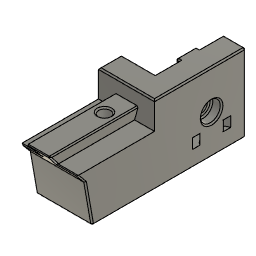
Support_arm_mount_Endcap_f360_v1 (Autodesk Fusion 360 design; units mm, degrees)
Autodesk Fusion 360 part; units mm, degrees
note: some values were not read from the file. Set by a fixed rule: which sketch regions a step uses.
sketch "Left" plane through (0, 0, 0) normal (1, 0, 0) x (0, 1, 0)
  line L0 (0, 0) -> (-50, 0)
  line L1 (-50, 0) -> (-50, 23)
  line L2 (-50, 23) -> (0, 23)
  line L3 (0, 23) -> (0, 0)
  line L4 (-50, 23) -> (-27, 23)
  line L5 (-27, 23) -> (-27, 15)
  line L6 (-27, 15) -> (-50, 15)
  line L7 (-50, 15) -> (-50, 23)
  line L8 (0, 0) -> (-20.2, 0)
  line L9 (-20.2, 0) -> (-20.2, 23)
  line L10 (-20.2, 23) -> (0, 23)
  line L11 (0, 23) -> (0, 0)
  circle A0 centre (-10.1, 11.5) radius 1.75
  line L12 (0, 0) -> (-10.1, 0) construction
  line L13 (-10.1, 0) -> (-10.1, 11.5) construction
  line L14 (-10.1, 11.5) -> (0, 11.5) construction
  line L15 (0, 11.5) -> (0, 0) construction
  circle A1 centre (-10.1, 11.5) radius 2.95
  line L16 (0, 0) -> (-20.2, 0)
  line L17 (-7.1, 0) -> (-13.1, 0)
  line L18 (-13.1, 0) -> (-13.1, 23)
  line L19 (-7.1, 0) -> (-7.1, 23)
  line L20 (-50, 15) -> (-37.4135, 0)
  line L21 (-50, 15) -> (-27, 15) construction
  line L22 (-50, 15) -> (-59.876, 26.7698)
  line L23 (-50, 0) -> (-56.7128, 0)
  line L24 (-56.7128, 0) -> (-56.7128, 23)
  line L25 (-56.7128, 23) -> (-50, 23)
  line L26 (-50, 23) -> (-50, 0)
  circle A2 centre (-45.4135, 6) radius 6
  circle A3 centre (-45.4135, 6) radius 4
  line L27 (-45.4135, 6) -> (-41.5568, 10.5963) construction
  line L28 (-45.4135, 6) -> (-41.4135, 6) construction
  line L29 (-41.5568, 10.5963) -> (-43.2297, 12)
  line L30 (-45.4135, 6) -> (-45.4135, 12) construction
  line L31 (-45.4135, 12) -> (-43.2297, 12)
  line L32 (-45.4135, 6) -> (-42.3493, 3.4288) construction
  line L33 (-42.3493, 3.4288) -> (-41.4135, 4.5441)
  line L34 (-41.4135, 6) -> (-41.4135, 4.5441)
  line L35 (-45.4135, 6) -> (-45.4135, 0)
  line L36 (-45.4135, 0) -> (-37.4135, 0)
  line L37 (-56.7128, 23) -> (-56.7128, 27) construction
  line L38 (-56.7128, 27) -> (-63.2177, 27) construction
  line L39 (-50, 15) -> (-50, 19) construction
  line L40 (-50, 19) -> (-53.3564, 19) construction
  line L41 (-45.4135, 0) -> (-49.469, 23)
  line L42 (-45.4135, 0) -> (-18.876, 0) construction
  point P0 (-10.1, 0)
  dimension "d1" = 50
  dimension "d2" = 23
  dimension "d3" = 23
  dimension "d4" = 8
  dimension "d5" = 20.2
  dimension "d6" = 23
  dimension "d7" = 10.1
  dimension "d8" = 11.5
  dimension "d9" = 3.5
  dimension "d10" = 5.9
  dimension "d11" = 6
  dimension "d12" = 180
  dimension "d13" = 50
  dimension "d47" = 12
  dimension "d48" = -2
  dimension "d49" = 50
  dimension "d50" = 8
  dimension "d51" = 6
  dimension "d64" = 4
  dimension "d65" = 4
  dimension "d66" = 100
  constraint horizontal L0
  constraint vertical L1
  constraint horizontal L2
  constraint vertical L3
  constraint coincident L0.start L3.end
  constraint horizontal L4
  constraint vertical L5
  constraint horizontal L6
  constraint vertical L7
  constraint horizontal L8
  constraint vertical L9
  constraint horizontal L10
  constraint vertical L11
  constraint horizontal L12
  constraint vertical L13
  constraint horizontal L14
  constraint vertical L15
  constraint coincident A0.centre L13.end
  constraint horizontal L17
  constraint coincident P0 L12.end
  constraint midpoint L17 P0
  constraint vertical L18
  constraint coincident L2 L18.end
  constraint coincident L10 L19.end
  constraint horizontal L21
  constraint coincident L0 L20.end
  constraint parallel L20 L22
  constraint horizontal L23
  constraint vertical L24
  constraint horizontal L25
  constraint vertical L26
  constraint coincident L22 L24.end
  constraint horizontal L28
  constraint coincident A2.centre A3.centre
  constraint coincident A2 L27.end
  constraint tangent A2 L29
  constraint coincident A2 L30.end
  constraint perpendicular L28 L30
  constraint tangent A2 L31
  constraint coincident A3 L32.end
  constraint perpendicular L27 L32
  constraint tangent A3 L33
  constraint coincident A3 L28.end
  constraint tangent A3 L34
  constraint coincident L0 L35.end
  constraint perpendicular L0 L35
  constraint perpendicular L25 L37
  constraint perpendicular L37 L38
  constraint perpendicular L6 L39
  constraint coincident L22 L40.end
  constraint perpendicular L39 L40
  constraint horizontal L42
  constraint coincident L2 L41.end
  measures "d1" distance of L0.start L0.end
  measures "d2" distance of L0.start L2.end
  measures "d3" distance of L1.end L4.end
  measures "d4" distance of L4.end L5.end
  measures "d5" distance of L0.start L8.end
  measures "d6" distance of L0.start L2.end
  measures "d7" distance of A0.centre L14.end
  measures "d8" distance of P0 A0.centre
  measures "d9" diameter of A0
  measures "d10" diameter of A1
  measures "d11" distance of L17.start L17.end
  measures "d12" angle of L18 L19
  measures "d13" angle of L20 L21
  measures "d47" diameter of A2
  measures "d49" angle of L27 L28
  measures "d50" distance of L20.end L35.end
  measures "d51" distance of A2.centre L35.end
  measures "d64" distance of L24.end L37.end
  measures "d65" distance of L6.end L39.end
  measures "d66" angle of L41 L42
extrude "Extrude1" add sketch "Left" along normal mid plane 16.6 contours L0 L2 L3 L8 L10 L11 L16 L19 | L0 L2 L8 L10 L16 L17 L18 L19 | L0 L2 L8 L9 L10 L16 L18 | L0 L2 L5 L6 L9 L20 A2 L29 L31 L41 | L0 L20 A2 L36 | L20 A2 A3 L33 L34 L35 | A3 L35 L41 | L20 A2 A3 L34 | L20 A3 L41 | L20 A3 L33 L34 | L20 A3 L34 | L20 A2 A3 L41 | L20 A3 | A2 L29 L31 | L6 L20 L41 | L20 A2 L41 | A1
extrude "Extrude2" cut sketch "Left" against normal blind 3 from surface at 8.3 contours A0 | A1
extrude "Extrude3" cut sketch "Left" along normal blind 10 from surface at -8.3 contours L0 L2 L3 L8 L10 L11 L16 L19 | L0 L2 L8 L10 L16 L17 L18 L19 | L0 L2 L8 L9 L10 L16 L18 | A0 | A1
extrude "Extrude4" add sketch "Left" against normal blind 1 from surface at 1.7 contours L0 L2 L8 L10 L16 L17 L18 L19 | A1
sketch "Front" plane through (0, 0, 0) normal (0, 1, 0) x (1, 0, 0)
  line L0 (-8.3, -15) -> (8.3, -15)
  line L1 (8.3, -15) -> (8.3, -23)
  line L2 (8.3, -23) -> (-8.3, -23)
  line L3 (-8.3, -23) -> (-8.3, -15)
  line L4 (-2.4, -15) -> (2.4, -15)
  line L5 (0, -15) -> (0, -19) construction
  line L6 (-3.5, -19) -> (3.5, -19)
  line L7 (2.4, -15) -> (3.5, -19)
  line L8 (-2.4, -15) -> (-3.5, -19)
  dimension "d25" = 4.8
  dimension "d26" = 4
  dimension "d27" = 7
  constraint parallel L0 L4
  constraint midpoint L0 L5.start
  constraint perpendicular L0 L5
  constraint horizontal L6
  constraint midpoint L5.end L6
  constraint midpoint L4 L5.start
  measures "d25" distance of L4.start L4.end
  measures "d26" distance of L5.start L5.end
  measures "d27" distance of L6.start L6.end
extrude "Extrude5" add sketch "Front" against normal blind 28 from surface at -27 contours L0 L4 L6 L7 L8
extrude "Extrude6" cut sketch "Left" along normal mid plane 20 contours L1 L22 L23 L24 L26 A2 | L1 L26 A2
sketch "Top" plane through (0, 0, 0) normal (0, 0, 1) x (1, 0, 0)
  line L0 (-3.5, -50) -> (-3.5, -53.3564)
  line L1 (-3.5, -53.3564) -> (3.5, -53.3564)
  line L2 (3.5, -50) -> (3.5, -53.3564)
  line L3 (3.5, -50) -> (8.3, -50)
  line L4 (1.7, -7.1) -> (0.7, -7.1)
  line L5 (1.7, -13.1) -> (0.7, -13.1)
  line L6 (0.7, -7.1) -> (0.7, -13.1)
  line L7 (1.7, -20.2) -> (1.7, -13.1)
  line L8 (-8.3, -20.2) -> (1.7, -20.2)
  line L9 (1.7, -7.1) -> (1.7, 0)
  line L10 (-8.3, -20.2) -> (-8.3, -45.4135)
  line L11 (-8.3, -47.5419) -> (-8.3, -50)
  line L12 (1.7, 0) -> (8.3, 0)
  line L13 (8.3, -45.4135) -> (8.3, 0)
  line L14 (8.3, -50) -> (8.3, -47.5419)
  line L15 (-8.3, -50) -> (-3.5, -50)
  line L16 (8.3, -20.2) -> (-8.3, -20.2) construction
  line L17 (8.3, -50) -> (-8.3, -50) construction
  circle A0 centre (0, -33.5) radius 1.75
  circle A1 centre (0, -33.5) radius 2.9
  line L18 (0, -20.2) -> (0, -33.5) construction
  line L19 (0, -30.6) -> (-2.9, -33.5)
  line L20 (-2.9, -33.5) -> (0, -36.4)
  line L21 (0, -36.4) -> (2.9, -33.5)
  line L22 (2.9, -33.5) -> (0, -30.6)
  circle A2 centre (10.3, -10.1) radius 6
  circle A3 centre (10.3, -10.1) radius 4
  line L23 (8.3, 0) -> (8.3, -20.2)
  line L24 (8.3, -10.1) -> (10.3, -10.1) construction
  line L25 (-8.3, -45.4135) -> (-8.3, -47.5419)
  line L26 (8.3, -47.5419) -> (8.3, -45.4135)
  line L27 (0, -50) -> (-0.1825, -40.75) construction
  circle A4 centre (-0.1825, -40.75) radius 1.75
  circle A5 centre (-0.1825, -40.75) radius 2.45
  point P0 (0, -33.5)
  point P1 (0, -33.5)
  dimension "d36" = 3.5
  dimension "d37" = 5.8
  dimension "d39" = 13.3
  dimension "d54" = 12
  dimension "d55" = -2
  dimension "d56" = 2
  dimension "d67" = 9.25
  dimension "d68" = 3.5
  dimension "d69" = 4.9
  constraint coincident L13 L16.start
  constraint perpendicular L10 L16
  constraint coincident L8.start L10.start
  constraint coincident L3.end L14.start
  constraint coincident L11.end L15.start
  constraint coincident P1 P0
  constraint midpoint L16 L18.start
  constraint perpendicular L16 L18
  constraint coincident A1 L19.start
  constraint coincident L18 L19.start
  constraint coincident L12.end L13.end
  constraint midpoint L23 L24.start
  constraint perpendicular L23 L24
  constraint coincident A2.centre A3.centre
  constraint midpoint L17 L27.start
  constraint coincident L27.end A4.centre
  constraint concentric A4 A5
  measures "d36" diameter of A0
  measures "d37" diameter of A1
  measures "d39" distance of L18.start P1
  measures "d54" diameter of A2
  measures "d56" distance of L24.start A2.centre
  measures "d67" vertical distance of L27.start L27.end
  measures "d68" diameter of A4
  measures "d69" diameter of A5
extrude "Extrude7" cut sketch "Top" along normal blind 7 contours A0 | A1 L22 | A1 L21 | L19 L20 L21 L22 | A1 L19 | A1 L20
extrude "Extrude8" cut sketch "Top" along normal blind 0.2 from surface at 7 contours A0 | L19 L20 L21 L22
extrude "Extrude9" cut sketch "Top" along normal blind 25 contours A0
extrude "Extrude11" cut sketch "Top" along normal blind 3 from surface at 4.75 contours L13 A2 A3 L23 | L13 A2 A3 L23
extrude "Extrude12" cut sketch "Top" along normal blind 6.5 contours A4
extrude "Extrude13" cut sketch "Top" along normal blind 4 contours A5
chamfer "Chamfer1" distance 0.4 angle 45 17 edges at (8.3, 0, 11.5) (5.3, -12.8504, 12.5668) (8.3, -12.8504, 12.5668) (-1.6316, -32.8672, 19) (-2.7037, -34.5487, 0) (-8.3, -48.7709, 13.5353) (8.3, -48.7709, 13.5353) (5.35, -50, 15) (-5.35, -50, 15) (0, -53.3564, 19) (3.5, -40.1782, 19) (-3.5, -40.1782, 19) (-2.95, -51.6782, 17) (2.95, -51.6782, 17) (8.3, -46.4777, 6.0353) (-8.3, -46.4777, 6.0353) (-2.4667, -41.636, 4) 3 faces at (6.1, -13.3667, 23) (-2.5532, -23.7335, 0) (0.7, -10.0564, 3.2516)
